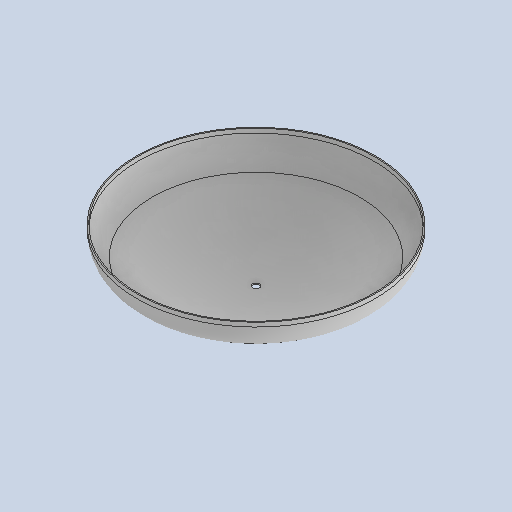
# Autodesk Inventor part: TZS 1208 dished head
Saved by Autodesk Inventor 2025 (Build 290162010, 162A)
## iProperties
Created: 2025-02-16
Part Number: TZS 1208 dished head
Material: Steel
Document SubType Name: Modeling
Designer: pokla
Density: 7.85 g/cm^3
Appearance: Default
Mass: 71183.4 g
Surface Area: 30460.9 cm^2
Volume: 9067.95 cm^3
Author: pokla
Autodesk Inventor part; units mm, degrees
ref_plane "YZ Plane" through (0, 0, 0) normal (1, 0, 0) x (0, 1, 0)
ref_plane "XZ Plane" through (0, 0, 0) normal (0, 1, 0) x (-1, 0, 0)
ref_plane "XY Plane" through (0, 0, 0) normal (0, 0, 1) x (1, 0, 0)
sketch "Sketch1" plane through (0, 0, 0) normal (0, 1, 0) x (-1, 0, 0)
  line L0 (600, 0) -> (600, -21)
  arc A0 (523.9158, -145.5583) -> (600, -21) centre (460, -21) ccw
  arc A1 (17.5, -272) -> (523.9158, -145.5583) centre (0, 875.442) ccw
  line L1 (0, 272) -> (0, -272)
  arc A2 (17.5, -265.9993) -> (521.1766, -140.2201) centre (0, 875.442) ccw
  arc A3 (521.1766, -140.2201) -> (594, -21) centre (460, -21) ccw
  line L2 (594, -21) -> (594, 0)
  line L3 (594, 0) -> (600, 0)
  line L4 (0, -272) -> (17.5, -272)
  line L5 (0, -265.9993) -> (17.5, -265.9993)
  line L6 (17.5, -272) -> (17.5, -265.9993)
  point P0 (0, 0)
  point P1 (0, 0)
  point P2 (0, -163.7009)
  point P3 (0, -169.7009)
  dimension "d0" = 140
  dimension "d1" = 21
  dimension "d3" = 1147.5754
  dimension "d6" = 6
  dimension "d13" = 35
  dimension "d14" = 1200
  dimension "d15" = 272
  constraints: 14 end point, 8 point on circle, 4 centre point, 2 horizontal, 2 parallel, 2 tangent, 2 vertical, 1 coincident, 1 horizontal alignment, 1 line through centre, 1 midpoint, 1 perpendicular, 1 point on line, 2 other
  measures "d0" radius of A0
  measures "d1" distance of L0.start L0.end
  measures "d3" radius of A1
  measures "d6" radial gap between concentric circles of A1 A2
  measures "d13" diameter of L4.end L1
  measures "d14" diameter of L0 L1
  measures "d15" distance of point (0, 0) L1.end
revolve "Revolution1" add sketch "Sketch1" angle 360 about axis through (0, 0, 272) along (0, 0, -1) contours L0 A0 A1 L6 A2 A3 L2 L3
equation "\"d0\" = tech_dishhead_small_rad"
equation "\"d1\" = tech_dishhead_edge_hight"
equation "\"d13\" = tech_dishhead_bottom_hole"
equation "\"d14\" = MAIN_filter_diam"
equation "\"d15\" = MAIN_dished_head_hight"
equation "\"tech_dishhead_small_rad\" = 140"
equation "\"tech_dishhead_edge_hight\" = 21"
equation "\"tech_dishhead_bottom_hole\" = 35"
equation "\"MAIN_filter_diam\" = 1200"
equation "\"MAIN_dished_head_hight\" = 272"
body "Solid1"
